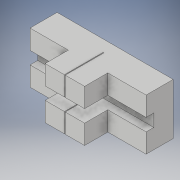
# Autodesk Inventor part: BalsaBoi
Saved by Autodesk Inventor 2018 (Build 220112000, 112)
## iProperties
Created: 2018-08-28
Part Number: BalsaBoi
Material: Generic
Document SubType Name: Modeling
Designer: F8PLTW
Density: 1 g/cm^3
Appearance: Default
Author: F8PLTW
Autodesk Inventor part; units mm, degrees
ref_plane "YZ Plane" through (0, 0, 0) normal (1, 0, 0) x (0, 1, 0)
ref_plane "XZ Plane" through (0, 0, 0) normal (0, 1, 0) x (-1, 0, 0)
ref_plane "XY Plane" through (0, 0, 0) normal (0, 0, 1) x (1, 0, 0)
sketch "Sketch1" plane through (0, 0, 0) normal (0, 0, 1) x (1, 0, 0)
  line L0 (-17.386, 3.6293) -> (12.614, 3.6293)
  line L1 (12.614, 3.6293) -> (12.614, -9.6107)
  line L2 (12.614, -9.6107) -> (-17.386, -9.6107)
  line L3 (-17.386, -9.6107) -> (-17.386, 3.6293)
  point P0 (0, 0)
  dimension "d0" = 30
  dimension "d1" = 13.24
  constraints: 8 end point, 2 parallel, 1 horizontal, 1 perpendicular
  measures "d0" distance of L1.end L2.end
  measures "d1" distance of L0.end L1.end
extrude "Extrusion1" add sketch "Sketch1" along normal blind 5
sketch "Sketch2" plane through (0, 0, 5) normal (0, 0, 1) x (1, 0, 0)
  line L0 (12.614, 3.6293) -> (-17.386, 3.6293) projected
  line L1 (-17.386, 3.6293) -> (-17.386, -9.6107) projected
  line L2 (12.614, 3.6293) -> (-17.386, 3.6293)
  line L3 (-17.386, 3.6293) -> (-17.386, -1.3707)
  line L4 (-17.386, -1.3707) -> (12.614, -1.3707)
  line L5 (12.614, -1.3707) -> (12.614, 3.6293)
  line L6 (12.614, -9.6107) -> (12.614, 3.6293) projected
  line L7 (-17.386, -9.6107) -> (12.614, -9.6107)
  line L8 (12.614, -9.6107) -> (12.614, -4.6107)
  line L9 (12.614, -4.6107) -> (-17.386, -4.6107)
  line L10 (-17.386, -4.6107) -> (-17.386, -9.6107)
  point P0 (0, 0)
  dimension "d4" = 5
  dimension "d5" = 5
  constraints: 16 end point, 4 parallel, 2 horizontal, 2 perpendicular, 2 point on line
  measures "d4" distance of L3.end L2.end
  measures "d5" distance of L8.end L7.end
extrude "Extrusion2" add sketch "Sketch2" along normal blind 2 contours L5 L4 L1 L0 | L6 L7 L1 L9
sketch "Sketch3" plane through (0, 0, 7) normal (0, 0, 1) x (1, 0, 0)
  line L0 (-2.386, 3.6293) -> (-2.386, -9.6107) construction
  line L1 (2.714, 3.6293) -> (-7.486, 3.6293)
  line L2 (-7.486, 3.6293) -> (-7.486, -1.3707)
  line L3 (-7.486, -1.3707) -> (2.714, -1.3707)
  line L4 (2.714, -1.3707) -> (2.714, 3.6293)
  line L5 (12.614, -2.9907) -> (-17.386, -2.9907) construction
  line L6 (2.714, -9.6107) -> (-7.486, -9.6107)
  line L7 (-7.486, -9.6107) -> (-7.486, -4.6107)
  line L8 (-7.486, -4.6107) -> (2.714, -4.6107)
  line L9 (2.714, -4.6107) -> (2.714, -9.6107)
  point P0 (0, 0)
  point P1 (12.614, -9.6107)
  point P2 (-17.386, -9.6107)
  dimension "d8" = 10.2
  constraints: 20 end point, 4 symmetric about line, 2 parallel, 1 horizontal, 1 perpendicular, 1 other
  measures "d8" distance of L3.end L2.end
extrude "Extrusion3" add sketch "Sketch3" along normal blind 6
sketch "Sketch4" plane through (0, 0, 13) normal (0, 0, 1) x (1, 0, 0)
  line L0 (2.714, 3.6293) -> (-7.486, 3.6293) projected
  line L1 (-2.386, 3.6293) -> (-2.386, -9.6107) construction
  line L2 (-7.486, -9.6107) -> (2.714, -9.6107) projected
  line L3 (-2.286, 3.6293) -> (-2.486, 3.6293)
  line L4 (-2.486, 3.6293) -> (-2.486, -9.6107)
  line L5 (-2.486, -9.6107) -> (-2.286, -9.6107)
  line L6 (-2.286, -9.6107) -> (-2.286, 3.6293)
  point P0 (0, 0)
  dimension "d11" = 0.2
  constraints: 10 end point, 2 midpoint, 2 parallel, 2 point on line, 1 horizontal, 1 perpendicular, 1 other
  measures "d11" distance between parallel lines of L4 L6
extrude "Extrusion4" cut sketch "Sketch4" against normal blind 10
body "Solid1"
